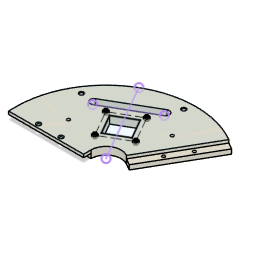
2nd_floor (Autodesk Fusion 360 design; units mm, degrees)
Autodesk Fusion 360 part; units mm, degrees
note: some values were not read from the file. Set by a fixed rule: which sketch regions a step uses.
sketch "Sketch1" plane through (0, 0, 0) normal (0, 1, 0) x (1, 0, 0)
  line L0 (-120, 0) -> (-20, 0)
  line L1 (10, 17.3205) -> (60, 103.923)
  arc A0 (60, 103.923) -> (-120, 0) centre (0, 0) ccw
  arc A1 (10, 17.3205) -> (-20, 0) centre (0, 0) ccw
  dimension "d57" = 240
  dimension "d58" = 120
  dimension "d59" = 40
  constraint coincident A0.centre A1.centre
  constraint horizontal L0
  constraint coincident L0 A0.centre
  constraint coincident A0.centre L1
  measures "d57" diameter of A0
  measures "d58" angle of L0 L1
  measures "d59" diameter of A1
extrude "Extrude3" add sketch "Sketch1" along normal blind 10
sketch "Sketch9" plane through (0, 0, 0) normal (0, 0, 1) x (1, 0, 0)
  line L0 (-120, 0) -> (-20, 0)
  line L1 (-20, 0) -> (-20, 10)
  line L2 (-20, 10) -> (-120, 10)
  line L3 (-120, 10) -> (-120, 0)
  line L4 (-120, 10) -> (-10, 10)
  line L5 (-10, 10) -> (-10, 6)
  line L6 (-10, 6) -> (-120, 6)
  line L7 (-120, 6) -> (-120, 10)
  dimension "d60" = 4
  constraint horizontal L4
  constraint vertical L5
  constraint horizontal L6
  constraint vertical L7
  constraint coincident L2.end L3.start
  measures "d60" distance of L2.end L6.end
extrude "Extrude8" add sketch "Sketch9" along normal blind 10 contours L1 L2 L3 L4 L6 L7
sketch "Sketch12" plane through (0, 0, 0) normal (0.866025, 0, 0.5) x (0.5, 0, -0.866025)
  line L0 (20, 0) -> (120, 0)
  line L1 (120, 0) -> (120, 10)
  line L2 (120, 10) -> (20, 10)
  line L3 (20, 10) -> (20, 0)
  line L4 (20, 0) -> (130, 0)
  line L5 (130, 0) -> (130, 6)
  line L6 (130, 6) -> (20, 6)
  line L7 (20, 6) -> (20, 0)
  dimension "d63" = 6
  constraint horizontal L4
  constraint vertical L5
  constraint horizontal L6
  constraint vertical L7
  constraint coincident L0.start L3.end
  measures "d63" distance of L0.start L6.end
extrude "Extrude9" add sketch "Sketch12" along normal blind 10 contours L0 L1 L3 L4 L6 L7
sketch "Sketch13" plane through (0, 10, 0) normal (0, 1, 0) x (-1, 0, 0)
  arc A0 (-60, -103.923) -> (120, 0) centre (0, 0) ccw
  arc A1 (-10, -17.3205) -> (20, 0) centre (0, 0) ccw
  line L0 (-10, -17.3205) -> (-60, -103.923)
  line L1 (120, 0) -> (120, 10)
  line L2 (120, 10) -> (20, 10)
  line L3 (20, 10) -> (20, 0)
  point P0 (85, 5)
  point P1 (55, 5)
  dimension "d178" = 30
  dimension "d179" = 35
  measures "d178" distance of P0 P1
  measures "d179" distance of P0 L1
hole "Hole1" at (-85, 10, 5) at (-55, 10, 5) direction (0, -1, 0) diameter 4 depth 4 tip angle 118 countersink diameter 6 countersink angle 90
sketch "Sketch14" plane through (0, 6, 0) normal (0, 1, 0) x (-1, 0, 0)
  line L0 (-60, -103.923) -> (-10, -17.3205)
  line L1 (-10, -17.3205) -> (-18.6603, -12.3205)
  line L2 (-18.6603, -12.3205) -> (-68.6603, -98.923)
  line L3 (-68.6603, -98.923) -> (-60, -103.923)
  line L4 (-14.3301, -14.8205) -> (-64.3301, -101.423) construction
  point P0 (-31.8301, -45.1314)
  point P1 (-46.8301, -71.1122)
  dimension "d75" = 35
  dimension "d76" = 35
  constraint midpoint L1 L4.start
  constraint midpoint L3 L4.end
  constraint coincident L4 P0
  constraint coincident L4 P1
  measures "d75" distance of L1 P0
  measures "d76" distance of L3 P1
hole "Hole2" at (31.8301, 6, -45.1314) at (46.8301, 6, -71.1122) direction (0, -1, 0) diameter 4 depth 15 tip angle 118
sketch "Sketch15" plane through (0, 10, 0) normal (0, 1, 0) x (-1, 0, 0)
  arc A0 (-60, -103.923) -> (120, 0) centre (0, 0) ccw
  arc A1 (-10, -17.3205) -> (20, 0) centre (0, 0) ccw
  line L0 (-10, -17.3205) -> (-60, -103.923)
  line L1 (0, 0) -> (60, -103.923) construction
  line L2 (20, 0) -> (120, 0)
  line L3 (56.6506, -48.1218) -> (13.3494, -73.1218) construction
  line L4 (57.1962, -87.0666) -> (46.8038, -93.0666) construction
  circle A2 centre (85, 5) radius 3
  circle A3 centre (55, 5) radius 3
  line L5 (120, 0) -> (120, 10)
  line L6 (120, 10) -> (20, 10)
  line L7 (20, 10) -> (20, 0)
  dimension "d80" = 60
  dimension "d81" = 50
  dimension "d82" = 25
  dimension "d83" = 50
  dimension "d95" = 6
  dimension "d96" = 12
  dimension "d97" = 34
  constraint coincident A0.centre A1.centre
  constraint coincident A0 L1.end
  constraint perpendicular L1 L3
  constraint perpendicular L1 L4
  measures "d80" angle of L1 L2
  measures "d81" distance of L3.start L3.end
  measures "d82" distance of L1 L3.end
  measures "d83" distance of L1.end L3
  measures "d95" distance of L1 L4.start
  measures "d96" distance of L4.start L4.end
  measures "d97" distance of L3 L4
sketch "Sketch16" plane through (0, 10, 0) normal (0, 1, 0) x (-1, 0, 0)
  line L0 (120, 0) -> (120, 10)
  line L1 (20, 0) -> (20, 10)
  line L2 (-10, -17.3205) -> (-18.6603, -12.3205)
  line L3 (-60, -103.923) -> (-68.6603, -98.923)
  line L4 (120, 5) -> (20, 5) construction
  line L5 (-14.3301, -14.8205) -> (-64.3301, -101.423) construction
  line L6 (-11.0289, -109.1025) -> (-97.6314, -59.1025) construction
  line L7 (100, -45) -> (100, 55) construction
  dimension "d98" = 100
  dimension "d99" = 50
  dimension "d100" = 20
  dimension "d101" = 20
  dimension "d102" = 100
  dimension "d103" = 50
  constraint midpoint L0 L4.start
  constraint midpoint L1 L4.end
  constraint midpoint L2 L5.start
  constraint midpoint L3 L5.end
  constraint vertical L7
  constraint perpendicular L5 L6
  measures "d98" distance of L6.start L6.end
  measures "d99" distance of L5 L6.start
  measures "d100" distance of L3 L6
  measures "d101" distance of L0 L7
  measures "d102" distance of L7.start L7.end
  measures "d103" distance of L4 L7.start
sketch "Sketch17" plane through (0, 0, 0) normal (0, -1, 0) x (1, 0, 0)
  circle A0 centre (31.8301, -45.1314) radius 2
  circle A1 centre (46.8301, -71.1122) radius 2
  arc A2 (-120, 0) -> (60, -103.923) centre (0, 0) ccw
  line L0 (60, -103.923) -> (68.6603, -98.923)
  line L1 (68.6603, -98.923) -> (18.6603, -12.3205)
  line L2 (18.6603, -12.3205) -> (10, -17.3205)
  arc A3 (-20, 0) -> (10, -17.3205) centre (0, 0) ccw
  line L3 (-20, 0) -> (-120, 0)
sketch "Sketch18" plane through (0, 0, 0) normal (0, -1, 0) x (1, 0, 0)
  point P0 (-100, -45)
  point P1 (11.0289, -109.1025)
  point P2 (-100, -45)
  point P3 (11.0289, -109.1025)
  constraint coincident P2 P0
  constraint coincident P3 P1
sketch "Sketch23" plane through (0, 10, 0) normal (0, 1, 0) x (-1, 0, 0)
  arc A0 (-60, -103.923) -> (120, 0) centre (0, 0) ccw
  arc A1 (-10, -17.3205) -> (20, 0) centre (0, 0) ccw
  line L0 (0, 0) -> (60, -103.923) construction
  line L1 (91.8013, -59.0045) -> (5.1987, -109.0045) construction
  line L2 (15.6891, -97.1743) -> (76.3109, -62.1743)
  arc A2 (76.3109, -62.1743) -> (71.3109, -53.5141) centre (73.8109, -57.8442) ccw
  line L3 (71.3109, -53.5141) -> (10.6891, -88.5141)
  arc A3 (10.6891, -88.5141) -> (15.6891, -97.1743) centre (13.1891, -92.8442) ccw
  line L4 (13.1891, -92.8442) -> (73.8109, -57.8442) construction
  circle A4 centre (85, 5) radius 3
  circle A5 centre (55, 5) radius 3
  line L5 (120, 0) -> (120, 10)
  line L6 (120, 10) -> (20, 10)
  line L7 (20, 10) -> (20, 0)
  dimension "d147" = 35
  dimension "d148" = 70
  dimension "d149" = 5
  dimension "d150" = 82
  dimension "d184" = 100
  dimension "d185" = 50
  dimension "d186" = 97
  dimension "d187" = 109.1284
  constraint coincident A0.centre A1.centre
  constraint midpoint A0 L0.end
  constraint perpendicular L0 L1
  constraint tangent L2 A2
  constraint tangent A2 L3
  constraint parallel L2 L3
  constraint tangent L3 A3
  constraint tangent L2 A3
  constraint perpendicular L0 L4
  measures "d147" distance of L0 A3.centre
  measures "d148" distance of A3.centre A2.centre
  measures "d149" distance of L2 L4
  measures "d150" distance of A0.centre L3
  measures "d184" distance of L1.start L1.end
  measures "d185" distance of L0 L1.start
  measures "d186" distance of A0.centre L1
  measures "d187" distance of A0.centre L1.start
hole "Hole5" at (-91.8013, 10, -59.0045) at (-5.1987, 10, -109.0045) direction (0, -1, 0) diameter 4.5 depth 42.794 tip angle 180 countersink diameter 6 countersink angle 90
extrude "Extrude15" cut sketch "Sketch23" against normal blind 150 contours L2 A2 L3 A3
sketch "Sketch24" plane through (0, 0, 0) normal (0, -1, 0) x (1, 0, 0)
  line L0 (-15.6891, -97.1743) -> (-76.3109, -62.1743)
  arc A0 (-71.3109, -53.5141) -> (-76.3109, -62.1743) centre (-73.8109, -57.8442) ccw
  line L1 (-71.3109, -53.5141) -> (-10.6891, -88.5141)
  arc A1 (-15.6891, -97.1743) -> (-10.6891, -88.5141) centre (-13.1891, -92.8442) ccw
  circle A2 centre (-91.8013, -59.0045) radius 2.25
  circle A3 centre (-5.1987, -109.0045) radius 2.25
  circle A4 centre (31.8301, -45.1314) radius 2
  circle A5 centre (46.8301, -71.1122) radius 2
  arc A6 (-120, 0) -> (60, -103.923) centre (0, 0) ccw
  line L2 (60, -103.923) -> (68.6603, -98.923)
  line L3 (68.6603, -98.923) -> (18.6603, -12.3205)
  line L4 (18.6603, -12.3205) -> (10, -17.3205)
  arc A7 (-20, 0) -> (10, -17.3205) centre (0, 0) ccw
  line L5 (-20, 0) -> (-120, 0)
  line L6 (10, -17.3205) -> (60, -103.923) construction
  line L7 (0, 0) -> (-70, 0) construction
  line L8 (0, 0) -> (35, -60.6218) construction
  line L9 (35, -60.6218) -> (17.6795, -70.6218) construction
  line L10 (-70, 0) -> (-70, -20) construction
  dimension "d153" = 70
  dimension "d154" = 70
  dimension "d155" = 20
  dimension "d161" = 20
  constraint coincident A6.centre A7.centre
  constraint parallel L5 L7
  constraint parallel L6 L8
  constraint perpendicular L8 L9
  constraint perpendicular L7 L10
  measures "d153" distance of A6.centre L7.end
  measures "d154" distance of A6.centre L8.end
  measures "d155" distance of L8.end L9.end
  measures "d161" distance of L7.end L10.end
hole "Hole6" at (17.6795, 0, -70.6218) at (-70, 0, -20) direction (0, 1, 0) diameter 4 depth 42.794 tip angle 180 countersink diameter 6 countersink angle 90
sketch "Sketch25" plane through (0, 10, 0) normal (0, 1, 0) x (-1, 0, 0)
  circle A0 centre (-17.6795, -70.6218) radius 2
  circle A1 centre (70, -20) radius 2
  line L0 (76.3109, -62.1743) -> (15.6891, -97.1743)
  arc A2 (10.6891, -88.5141) -> (15.6891, -97.1743) centre (13.1891, -92.8442) ccw
  line L1 (10.6891, -88.5141) -> (71.3109, -53.5141)
  arc A3 (76.3109, -62.1743) -> (71.3109, -53.5141) centre (73.8109, -57.8442) ccw
  circle A4 centre (91.8013, -59.0045) radius 3
  circle A5 centre (5.1987, -109.0045) radius 3
  circle A6 centre (85, 5) radius 3
  circle A7 centre (55, 5) radius 3
  arc A8 (-60, -103.923) -> (120, 0) centre (0, 0) ccw
  line L2 (120, 0) -> (120, 10)
  line L3 (120, 10) -> (20, 10)
  line L4 (20, 10) -> (20, 0)
  arc A9 (-10, -17.3205) -> (20, 0) centre (0, 0) ccw
  line L5 (-10, -17.3205) -> (-60, -103.923)
  line L6 (54.3205, -54.0859) -> (19.6795, -74.0859) construction
  line L7 (19.6795, -74.0859) -> (-0.3205, -39.4449) construction
  line L8 (-0.3205, -39.4449) -> (34.3205, -19.4449) construction
  line L9 (34.3205, -19.4449) -> (54.3205, -54.0859) construction
  line L10 (0, 0) -> (60, -103.923)
  line L11 (71.3109, -53.5141) -> (10.6891, -88.5141)
  line L12 (47.4904, -52.2558) -> (21.5096, -67.2558)
  line L13 (21.5096, -67.2558) -> (6.5096, -41.275)
  line L14 (6.5096, -41.275) -> (32.4904, -26.275)
  line L15 (32.4904, -26.275) -> (47.4904, -52.2558)
  point P0 (54.3205, -54.0859)
  point P1 (34.3205, -19.4449)
  point P2 (-0.3205, -39.4449)
  point P3 (19.6795, -74.0859)
  dimension "d162" = 40
  dimension "d163" = 40
  dimension "d164" = 20
  dimension "d165" = 8
  dimension "d169" = 5
  dimension "d170" = 5
  dimension "d172" = 5
  dimension "d173" = 5
  constraint parallel L1 L6
  constraint perpendicular L6 L7
  constraint perpendicular L7 L8
  constraint perpendicular L6 L9
  constraint coincident P0 L6.start
  constraint coincident P1 L8.end
  constraint coincident P2 L7.end
  constraint coincident P3 L6.end
  constraint parallel L6 L12
  constraint perpendicular L12 L13
  constraint perpendicular L10 L14
  constraint perpendicular L12 L15
  measures "d162" distance of P1 P0
  measures "d163" distance of P2 P1
  measures "d164" distance of L9 L10
  measures "d165" distance of L6 L11
  measures "d169" distance of L9 L15
  measures "d170" distance of L6 L12
  measures "d172" distance of L7 L13
  measures "d173" distance of L8 L14
hole "Hole7" at (-54.3205, 10, -54.0859) at (-34.3205, 10, -19.4449) at (0.3205, 10, -39.4449) at (-19.6795, 10, -74.0859) direction (0, -1, 0) diameter 4 depth 20 tip angle 118
extrude "Extrude16" cut sketch "Sketch25" against normal blind 40 contours L10 L12 L13 L14 | L10 L12 L14 L15
equation "d82 = d81 / 2"
equation "d96 = d95 * 2"
equation "d99 = d98 / 2"
equation "d101 = d100"
equation "d102 = d98"
equation "d103 = d99"
equation "d148 = d147 * 2"
equation "d164 = d163 / 2"
equation "d185 = d184 / 2"
